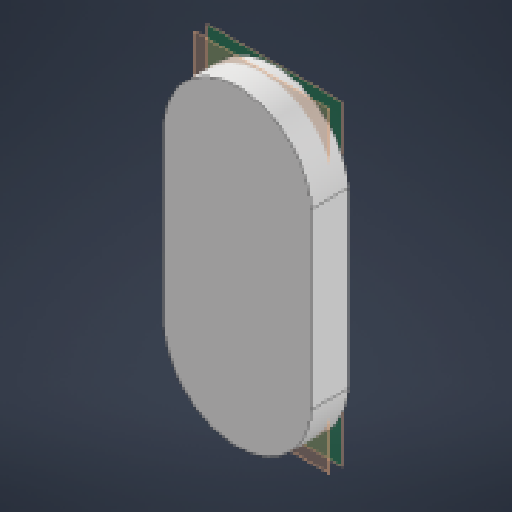
# Autodesk Inventor part: battery_case_top
Saved by Autodesk Inventor 2024 (Build 280153000, 153)
## iProperties
Created: 2026-08-20
Part Number: battery_case_top
Material: Generic
Document SubType Name: Modeling
Designer: schar
Density: 1 g/cm^3
Appearance: Default
Author: schar
Autodesk Inventor part; units mm, degrees
ref_plane "Work Plane1" through (0, 0, 0) normal (0, 0, 1) x (1, 0, 0)
sketch "Sketch1" plane through (0, 0, 0) normal (0, 0, 1) x (1, 0, 0)
  line L0 (119.8428, -136.5657) -> (119.8428, -115.4866) projected
  arc A0 (119.8428, -115.4866) -> (104.8622, -116.0261) centre (112.3622, -116.0261) ccw projected
  line L1 (104.8622, -136.0261) -> (104.8622, -116.0261) projected
  arc A1 (104.8622, -136.0261) -> (119.8428, -136.5657) centre (112.3622, -136.0261) ccw projected
  circle A2 centre (117.3428, -116.0541) radius 0.5 projected
  circle A3 centre (106.6428, -124.9791) radius 0.5 projected
  circle A4 centre (106.6428, -127.5191) radius 0.5 projected
  circle A5 centre (117.3428, -136.0541) radius 0.5 projected
  arc A6 (103.3319, -124.86) -> (103.3319, -127.1923) centre (106.6319, -126.0261) ccw projected
  line L2 (103.3319, -124.86) -> (103.3319, -116.0261) projected
  arc A7 (121.3731, -115.4341) -> (103.3319, -116.0261) centre (112.3622, -116.0261) ccw projected
  line L3 (121.3731, -115.4341) -> (121.3731, -136.6182) projected
  arc A8 (103.3319, -136.0261) -> (121.3731, -136.6182) centre (112.3622, -136.0261) ccw projected
  line L4 (103.3319, -136.0261) -> (103.3319, -127.1923) projected
  arc A9 (121.8731, -115.4179) -> (102.8319, -116.0261) centre (112.3622, -116.0261) ccw projected
  line L5 (102.8319, -116.0261) -> (102.8319, -136.0261) projected
  arc A10 (102.8319, -136.0261) -> (121.8731, -136.6344) centre (112.3622, -136.0261) ccw projected
  line L6 (121.8731, -136.6344) -> (121.8731, -115.4179) projected
  point P0 (0, 0)
  point P1 (107.9, -107.4721)
  point P2 (107.9, -127.4721)
extrude "Extrusion1" add sketch "Sketch1" along normal blind 3 contours A1 L1 A0 L0 | A2 | A3 | A4 | A5
ref_plane "Work Plane3" through (97.1697, -138.2024, -7.9168) normal (0, 0, 1) x (1, 0, 0)
ref_plane "Work Plane4" through (100.4, -134.9721, -1.51) normal (0, 0, -1) x (0, 1, 0)
sketch "Sketch4" plane through (0, 0, 3) normal (0, 0, 1) x (1, 0, 0)
  line L0 (103.3319, -124.86) -> (103.3319, -116.0261)
  line L1 (103.3319, -136.0261) -> (103.3319, -127.1923)
  arc A0 (103.3319, -136.0261) -> (121.3731, -136.6182) centre (112.3622, -136.0261) ccw
  line L2 (121.3731, -115.4341) -> (121.3731, -136.6182)
  arc A1 (121.3731, -115.4341) -> (103.3319, -116.0261) centre (112.3622, -116.0261) ccw
  line L3 (103.3319, -124.86) -> (103.3319, -127.1923)
  circle A2 centre (112.3622, -136.0261) radius 6.35
  line L4 (119.8428, -136.5657) -> (119.8428, -115.4866)
  arc A3 (119.8428, -115.4866) -> (104.8622, -116.0261) centre (112.3622, -116.0261) ccw
  line L5 (104.8622, -116.0261) -> (104.8622, -136.0261)
  arc A4 (104.8622, -136.0261) -> (119.8428, -136.5657) centre (112.3622, -136.0261) ccw
  point P0 (0, 0)
extrude "Extrusion4" add sketch "Sketch4" against normal up to surface (4.51 mm away) contours L0 A1 L2 A0 L1 L3
sketch "Sketch5" plane through (121.3731, -136.6182, -1.51) normal (0, 0, -1) x (-1, 0, 0)
  line L0 (16.5109, 20.5921) -> (16.5109, 13.6117) projected
  line L1 (16.5109, 0.5921) -> (16.5109, 20.5921) projected
  arc A0 (1.5303, 0.0526) -> (16.5109, 0.5921) centre (9.0109, 0.5921) ccw projected
  line L2 (1.5303, 0.0526) -> (1.5303, 21.1316) projected
  arc A1 (16.5109, 20.5921) -> (1.5303, 21.1316) centre (9.0109, 20.5921) ccw projected
  line L3 (1.3303, 21.1388) -> (1.3303, 0.0454)
  arc A2 (1.3303, 0.0454) -> (16.7109, 0.5921) centre (9.0109, 0.5921) ccw
  line L4 (16.7109, 0.5921) -> (16.7109, 20.5921)
  arc A3 (16.7109, 20.5921) -> (1.3303, 21.1388) centre (9.0109, 20.5921) ccw
  point P0 (121.3731, 136.6182)
  dimension "d10" = 0.2
  constraints: 4 end point, 4 point on circle, 2 centre point, 3 other
  measures "d10" distance between parallel lines of L2 L3
extrude "Extrusion5" cut sketch "Sketch5" against normal up to surface (1.51 mm away)
ref_plane "Work Plane5" through (93.9197, -138.2024, -7.9168) normal (0, 0, 1) x (1, 0, 0)
ref_plane "Work Plane6" through (93.9197, -138.2024, -7.9168) normal (0, 0, 1) x (1, 0, 0)
sketch "Sketch10" plane through (0, 0, 3) normal (0, 0, 1) x (1, 0, 0)
  line L0 (103.3319, -116.0261) -> (103.3319, -136.0261) projected
  arc A0 (103.3319, -124.86) -> (103.3319, -127.1923) centre (106.6319, -126.0261) ccw projected
  point P0 (0, 0)
  point P1 (103.3319, -135.2618)
extrude "Extrusion10" add sketch "Sketch10" against normal up to surface (4.51 mm away)
sketch "Sketch11" plane through (0, 0, 3) normal (0, 0, 1) x (1, 0, 0)
  circle A0 centre (124.0731, -115.3807) radius 1.5 projected
  circle A1 centre (100.6319, -116.0261) radius 1.5 projected
  circle A2 centre (124.0731, -136.6716) radius 1.5 projected
  circle A3 centre (100.6319, -136.0261) radius 1.5 projected
  line L0 (101.6319, -119.276) -> (100.632, -118.2761) projected
  line L1 (101.6319, -119.276) -> (101.6319, -132.7858) projected
  line L2 (101.6319, -132.7858) -> (100.6415, -133.7762) projected
  arc A4 (100.6415, -133.7762) -> (99.8748, -138.1449) centre (100.6319, -136.0261) ccw projected
  line L3 (99.8748, -138.1449) -> (102.4702, -140.1841) projected
  arc A5 (102.4702, -140.1841) -> (121.9777, -140.7888) centre (112.3622, -136.0261) ccw projected
  line L4 (124.6926, -138.8347) -> (121.9777, -140.7888) projected
  arc A6 (124.6926, -138.8347) -> (125.0601, -134.6496) centre (124.0731, -136.6716) ccw projected
  line L5 (125.0601, -134.6496) -> (123.0731, -132.4216) projected
  line L6 (123.0731, -132.4216) -> (123.0731, -119.6307) projected
  line L7 (125.0601, -117.4026) -> (123.0731, -119.6307) projected
  arc A7 (125.0601, -117.4026) -> (124.6926, -113.2176) centre (124.0731, -115.3807) ccw projected
  line L8 (124.6926, -113.2176) -> (121.9777, -111.2635) projected
  arc A8 (121.9777, -111.2635) -> (102.4702, -111.8682) centre (112.3622, -116.0261) ccw projected
  line L9 (99.8748, -113.9074) -> (102.4702, -111.8682) projected
  arc A9 (99.8748, -113.9074) -> (100.6319, -118.2761) centre (100.6319, -116.0261) ccw projected
  arc A10 (102.3319, -136.0261) -> (122.3731, -136.6502) centre (112.3622, -136.0261) ccw projected
  line L10 (102.3319, -136.0261) -> (102.3319, -116.0261) projected
  arc A11 (122.3731, -115.4021) -> (102.3319, -116.0261) centre (112.3622, -116.0261) ccw projected
  line L11 (122.3731, -115.4021) -> (122.3731, -136.6502) projected
  line L12 (102.3319, -136.0261) -> (102.3319, -116.0261) projected
  arc A12 (102.3319, -136.0261) -> (122.3731, -136.6502) centre (112.3622, -136.0261) ccw projected
  line L13 (122.3731, -115.4021) -> (122.3731, -136.6502) projected
  arc A13 (122.3731, -115.4021) -> (102.3319, -116.0261) centre (112.3622, -116.0261) ccw projected
  line L14 (102.8319, -116.0261) -> (102.8319, -136.0261) projected
  arc A14 (121.8731, -115.4179) -> (102.8319, -116.0261) centre (112.3622, -116.0261) ccw projected
  line L15 (121.8731, -136.6344) -> (121.8731, -115.4179) projected
  arc A15 (102.8319, -136.0261) -> (121.8731, -136.6344) centre (112.3622, -136.0261) ccw projected
  arc A16 (121.8731, -115.4179) -> (102.8319, -116.0261) centre (112.3622, -116.0261) ccw projected
  line L16 (102.8319, -116.0261) -> (102.8319, -136.0261) projected
  arc A17 (102.8319, -136.0261) -> (121.8731, -136.6344) centre (112.3622, -136.0261) ccw projected
  line L17 (121.8731, -136.6344) -> (121.8731, -115.4179) projected
  arc A18 (103.3319, -124.86) -> (103.3319, -127.1923) centre (106.6319, -126.0261) ccw projected
  line L18 (103.3319, -124.86) -> (103.3319, -116.0261) projected
  arc A19 (121.3731, -115.4341) -> (103.3319, -116.0261) centre (112.3622, -116.0261) ccw projected
  line L19 (121.3731, -115.4341) -> (121.3731, -136.6182) projected
  arc A20 (103.3319, -136.0261) -> (121.3731, -136.6182) centre (112.3622, -136.0261) ccw projected
  line L20 (103.3319, -136.0261) -> (103.3319, -127.1923) projected
  line L21 (101.6319, -119.276) -> (101.6319, -132.7858)
  line L22 (101.6319, -132.7858) -> (100.6415, -133.7762)
  circle A21 centre (100.6319, -136.0261) radius 2.25
  line L23 (99.8748, -138.1449) -> (102.4702, -140.1841)
  circle A22 centre (112.3622, -136.0261) radius 10.7303
  line L24 (121.9777, -140.7888) -> (124.6926, -138.8347)
  circle A23 centre (124.0731, -136.6716) radius 2.25
  line L25 (123.0731, -132.4216) -> (125.0601, -134.6496)
  line L26 (123.0731, -132.4216) -> (123.0731, -119.6307)
  line L27 (123.0731, -119.6307) -> (125.0601, -117.4026)
  line L28 (124.6926, -113.2176) -> (121.9777, -111.2635)
  circle A24 centre (112.3622, -116.0261) radius 10.7303
  line L29 (102.4702, -111.8682) -> (99.8748, -113.9074)
  circle A25 centre (100.6319, -116.0261) radius 2.25
  line L30 (100.6319, -118.2761) -> (101.6319, -119.276)
  circle A26 centre (124.0731, -115.3807) radius 2.25
  point P0 (0, 0)
  constraints: 20 end point, 6 coincident, 5 collinear, 1 centre point, 1 concentric, 1 point on line, 15 other
ref_plane "Work Plane8" through (98.3819, -146.7565, -7.9168) normal (0, 0, 1) x (1, 0, 0)
extrude "Extrusion11" add sketch "Sketch11" against normal up to surface (10.9168 mm away) contours A0 A24 A26 A7 | A0 A24 A26 L11 A11 | A26 A11 A25 A24 A8 | A24 L8 A26 | A26 L7 L6 L5 A23 A22 L11 A24 | A24 L11 A26 | A26 A14 A25 A11 | A11 L11 A26 L15 A14 | A24 L15 A26 L11 | L11 A22 L15 A24 | A24 A25 L9 | A25 A14 L14 L10 A11 | A11 L10 A25 A24 A1 | A26 L15 A24 L19 A19 L18 L14 A25 A14 | A14 L15 A26 | A22 A23 L11 | L11 A23 L15 A22 | L15 A22 L19 A24 | A25 A24 A1 A9 | A25 L14 A14 | A23 A22 A2 A10 L11 | L11 A10 A23 A15 L15 | A23 A6 A22 A2 | L15 A23 A15 A21 L14 A22 L20 A20 L19 | A25 A24 L10 A22 A21 L2 L1 L0 | A25 L14 A24 L10 | L10 A24 A25 | L15 A15 A23 | A24 L14 A22 L10 | A23 A22 A5 A21 A10 | A10 A21 A15 A23 | A22 L14 A21 L10 | L10 A21 A22 | A24 L18 A18 L20 A22 L14 | A21 A22 A3 L10 A10 | A10 L10 A21 L14 A15 | A23 L4 A22 | A15 L14 A21 | A21 A22 A3 A4 | A22 L3 A21
sketch "Sketch13" plane through (101.6319, -132.7858, -7.9168) normal (0, 0, -1) x (-1, 0, 0)
  line L0 (-1.7, 5.5934) -> (-1.7, -3.2404) projected
  line L1 (-1.7, 5.5934) -> (-1.7, 7.9258)
  arc A0 (-19.7412, -3.8325) -> (-1.7, -3.2404) centre (-10.7303, -3.2404) ccw projected
  line L2 (-19.7412, 17.3517) -> (-19.7412, -3.8325) projected
  arc A1 (-1.7, 16.7596) -> (-19.7412, 17.3517) centre (-10.7303, 16.7596) ccw projected
  line L3 (-1.7, 7.9258) -> (-1.7, 16.7596) projected
  line L4 (-1.2, -3.2404) -> (-1.2, 5.5934)
  line L5 (-1.2, 5.5934) -> (-1.2, 7.9258)
  line L6 (-1.2, 7.9258) -> (-1.2, 16.7596)
  arc A2 (-1.2, 16.7596) -> (-20.2412, 17.3679) centre (-10.7303, 16.7596) ccw
  line L7 (-20.2412, 17.3679) -> (-20.2412, -3.8486)
  arc A3 (-20.2412, -3.8486) -> (-1.2, -3.2404) centre (-10.7303, -3.2404) ccw
  line L8 (-0.7, 5.5934) -> (-0.7, -3.2404)
  arc A4 (-20.7412, -3.8644) -> (-0.7, -3.2404) centre (-10.7303, -3.2404) ccw
  line L9 (-20.7412, -3.8644) -> (-20.7412, 17.3837)
  arc A5 (-0.7, 16.7596) -> (-20.7412, 17.3837) centre (-10.7303, 16.7596) ccw
  line L10 (-0.7, 16.7596) -> (-0.7, 7.9258)
  line L11 (-0.7, 7.9258) -> (-0.7, 5.5934)
  point P0 (101.6319, 132.7858)
  dimension "d31" = 0.5
  dimension "d32" = 0.5
  constraints: 18 end point, 8 point on circle, 4 centre point, 1 vertical, 10 other
  measures "d31" distance between parallel lines of L0 L4
  measures "d32" distance between parallel lines of L4 L8
extrude "Extrusion12" cut sketch "Sketch13" against normal blind 1 contours L8 A4 L9 A5 L10 L11
fillet "Fillet4" radius 1 4 edges at (112.0298, -105.301, 3) (101.6319, -126.0309, 3) (112.0298, -146.7513, 3) (123.0731, -126.0261, 3)
body "Solid1"
